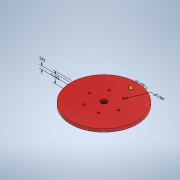
# Autodesk Inventor part: attachementToTripod
Saved by Autodesk Inventor 2022.2 (Build 262287010, 287A)
## iProperties
Created: 2021-02-15
Part Number: attachementToTripod
Material: PC/ABS Plastic
Document SubType Name: Modeling
Designer: robst
Density: 0.357273 g/cm^3
Appearance: Red
Author: robst
Autodesk Inventor part; units mm, degrees
(part 1 of 2)
ref_plane "YZ Plane" through (0, 0, 0) normal (1, 0, 0) x (0, 1, 0)
ref_plane "XZ Plane" through (0, 0, 0) normal (0, 1, 0) x (-1, 0, 0)
ref_plane "XY Plane" through (0, 0, 0) normal (0, 0, 1) x (1, 0, 0)
sketch "Sketch2" plane through (0, 0, 0) normal (0, 0, 1) x (1, 0, 0)
  line L0 (-101.6, 0) -> (-101.6, -9.525)
  line L1 (-101.6, -9.525) -> (-12.7, -9.525)
  line L2 (-10.795, -44.525) -> (0, -44.525)
  line L3 (-101.6, 0) -> (0, 0)
  line L4 (0, 0) -> (0, -44.525) construction
  line L5 (0, 0) -> (0, -44.525)
  line L6 (0, -53.43) -> (0, 8.905) projected
  line L7 (-12.7, -9.525) -> (-10.795, -44.525)
  dimension "d0" = 101.6
  dimension "d3" = 9.525
  dimension "d4" = 35
  dimension "d64" = 10.795
  constraints: 14 end point, 3 vertical, 2 horizontal, 1 perpendicular
  measures "d0" distance from line of L0 L3.end
  measures "d3" distance from line of L1 L3.end
  measures "d4" distance from line of L2.start L1
  measures "d64" horizontal distance of L2.start L3.end
revolve "Revolution1" add sketch "Sketch2" angle 360 about axis through (0, -10, 0) along (0, 1, 0)
sketch "Sketch5" plane through (0, -9.525, 0) normal (0, -1, 0) x (1, 0, 0)
  circle A0 centre (0, 0) radius 76.2 construction
  line L0 (-16.696, -77.6726) -> (-16.6474, -77.6818)
  spline S0 degree 2 poles (-16.6474, -77.6818) (-16.5292, -77.7545) (-16.0721, -77.9292) (-15.8841, -77.9649) knots 0 0 0 1 2 2 2
  spline S1 degree 2 poles (-15.8841, -77.9649) (-15.2895, -78.0777) (-14.6786, -77.6405) (-14.5451, -76.9367) knots 0 0 0 1 2 2 2
  line L1 (-14.5451, -76.9367) -> (-14.5094, -76.7486)
  line L2 (-14.5094, -76.7486) -> (-16.0747, -76.4517)
  line L3 (-16.0747, -76.4517) -> (-15.9262, -75.6691)
  line L4 (-15.9262, -75.6691) -> (-14.3913, -75.9603)
  line L5 (-14.3913, -75.9603) -> (-13.474, -71.125)
  line L6 (-13.474, -71.125) -> (-12.5276, -71.3045)
  line L7 (-12.5276, -71.3045) -> (-13.4449, -76.1398)
  line L8 (-13.4449, -76.1398) -> (-12.8078, -76.2606)
  line L9 (-12.8078, -76.2606) -> (-12.9563, -77.0433)
  line L10 (-12.9563, -77.0433) -> (-13.5933, -76.9224)
  line L11 (-13.5933, -76.9224) -> (-13.629, -77.1105)
  spline S2 degree 2 poles (-13.629, -77.1105) (-13.8201, -78.1176) (-14.9971, -78.9879) (-15.9071, -78.8153) knots 0 0 0 1 2 2 2
  spline S3 degree 2 poles (-15.9071, -78.8153) (-16.168, -78.7658) (-16.6612, -78.6157) (-16.8605, -78.5401) knots 0 0 0 1 2 2 2
  line L12 (-16.8605, -78.5401) -> (-16.696, -77.6726)
  line L13 (-16.8729, -70.3978) -> (-15.9346, -70.6161)
  line L14 (-15.9346, -70.6161) -> (-17.2303, -76.1854)
  line L15 (-17.2303, -76.1854) -> (-18.1686, -75.9671)
  line L16 (-18.1686, -75.9671) -> (-16.8729, -70.3978)
  line L17 (-18.4502, -76.878) -> (-17.3857, -77.1256)
  line L18 (-17.3857, -77.1256) -> (-17.6124, -78.1)
  line L19 (-17.6124, -78.1) -> (-18.6769, -77.8523)
  line L20 (-18.6769, -77.8523) -> (-18.4502, -76.878)
  line L21 (-19.193, -69.801) -> (-18.2625, -70.0502)
  line L22 (-18.2625, -70.0502) -> (-20.3217, -77.7388)
  line L23 (-20.3217, -77.7388) -> (-21.2522, -77.4896)
  line L24 (-21.2522, -77.4896) -> (-19.193, -69.801)
  spline S4 degree 2 poles (-22.8786, -68.5442) (-21.5758, -68.9706) (-20.6221, -70.9005) (-21.0639, -72.2503) knots 0 0 0 1 2 2 2
  spline S5 degree 2 poles (-21.0639, -72.2503) (-21.4979, -73.5767) (-23.4036, -74.6943) (-24.5245, -74.3274) knots 0 0 0 1 2 2 2
  spline S6 degree 2 poles (-24.5245, -74.3274) (-25.0292, -74.1622) (-25.7137, -73.6133) (-25.8995, -73.2082) knots 0 0 0 1 2 2 2
  spline S7 degree 2 poles (-25.8995, -73.2082) (-26.0911, -72.8011) (-26.1083, -71.8014) (-25.8951, -71.1499) knots 0 0 0 1 2 2 2
  line L25 (-25.8951, -71.1499) -> (-25.7318, -70.6511)
  line L26 (-25.7318, -70.6511) -> (-21.97, -71.8823)
  spline S8 degree 2 poles (-21.97, -71.8823) (-21.6607, -70.9374) (-22.283, -69.6227) (-23.1281, -69.3461) knots 0 0 0 1 2 2 2
  spline S9 degree 2 poles (-23.1281, -69.3461) (-23.4274, -69.2482) (-24.0526, -69.193) (-24.3219, -69.2218) knots 0 0 0 1 2 2 2
  spline S10 degree 2 poles (-24.3219, -69.2218) (-24.6068, -69.2585) (-25.0144, -69.3525) (-25.1567, -69.4099) knots 0 0 0 1 2 2 2
  line L27 (-25.1567, -69.4099) -> (-25.2095, -69.3926)
  line L28 (-25.2095, -69.3926) -> (-24.883, -68.395)
  spline S11 degree 2 poles (-24.883, -68.395) (-24.7034, -68.3823) (-24.1607, -68.352) (-23.9556, -68.3606) knots 0 0 0 1 2 2 2
  spline S12 degree 2 poles (-23.9556, -68.3606) (-23.6665, -68.3708) (-23.2073, -68.4366) (-22.8786, -68.5442) knots 0 0 0 1 2 2 2
  spline S13 degree 2 poles (-25.0684, -71.6414) (-25.1776, -72.015) (-25.2017, -72.6049) (-25.1146, -72.8348) knots 0 0 0 1 2 2 2
  spline S14 degree 2 poles (-25.1146, -72.8348) (-25.0233, -73.0921) (-24.5956, -73.4725) (-24.2258, -73.5935) knots 0 0 0 1 2 2 2
  spline S15 degree 2 poles (-24.2258, -73.5935) (-23.862, -73.7126) (-23.2803, -73.6625) (-22.9999, -73.5204) knots 0 0 0 1 2 2 2
  spline S16 degree 2 poles (-22.9999, -73.5204) (-22.7234, -73.3705) (-22.3412, -72.9173) (-22.1986, -72.5807) knots 0 0 0 1 2 2 2
  line L29 (-22.1986, -72.5807) -> (-25.0684, -71.6414)
  line L30 (-27.4155, -67.0006) -> (-26.28, -67.454)
  line L31 (-26.28, -67.454) -> (-26.8205, -68.8074)
  line L32 (-26.8205, -68.8074) -> (-27.956, -68.354)
  line L33 (-27.956, -68.354) -> (-27.4155, -67.0006)
  line L34 (-28.9957, -70.9575) -> (-27.8602, -71.4109)
  line L35 (-27.8602, -71.4109) -> (-28.4007, -72.7643)
  line L36 (-28.4007, -72.7643) -> (-29.5362, -72.3109)
  line L37 (-29.5362, -72.3109) -> (-28.9957, -70.9575)
  spline S17 degree 2 poles (-35.2717, -63.9178) (-35.1275, -63.8965) (-34.6336, -63.8095) (-34.4266, -63.8147) knots 0 0 0 1 2 2 2
  spline S18 degree 2 poles (-34.4266, -63.8147) (-34.1392, -63.8136) (-33.6527, -63.9114) (-33.2711, -64.1144) knots 0 0 0 1 2 2 2
  spline S19 degree 2 poles (-33.2711, -64.1144) (-32.9603, -64.2796) (-32.5234, -64.8127) (-32.4239, -65.1384) knots 0 0 0 1 2 2 2
  spline S20 degree 2 poles (-32.4239, -65.1384) (-32.3323, -65.4528) (-32.4117, -66.1939) (-32.5914, -66.532) knots 0 0 0 1 2 2 2
  spline S21 degree 2 poles (-32.5914, -66.532) (-32.8697, -67.0554) (-33.7056, -67.562) (-34.2985, -67.5196) knots 0 0 0 1 2 2 2
  spline S22 degree 2 poles (-34.2985, -67.5196) (-34.8281, -67.4897) (-36.0623, -67.0223) (-36.7532, -66.7038) knots 0 0 0 1 2 2 2
  line L38 (-36.7532, -66.7038) -> (-36.8401, -66.8674)
  spline S23 degree 2 poles (-36.8401, -66.8674) (-36.9967, -67.1618) (-37.011, -67.6228) (-36.9025, -67.8134) knots 0 0 0 1 2 2 2
  spline S24 degree 2 poles (-36.9025, -67.8134) (-36.7941, -68.0039) (-36.36, -68.3187) (-36.1092, -68.452) knots 0 0 0 1 2 2 2
  spline S25 degree 2 poles (-36.1092, -68.452) (-35.8148, -68.6086) (-34.926, -68.8574) (-34.4381, -68.9) knots 0 0 0 1 2 2 2
  line L39 (-34.4381, -68.9) -> (-34.389, -68.9261)
  line L40 (-34.389, -68.9261) -> (-34.85, -69.793)
  spline S26 degree 2 poles (-34.85, -69.793) (-35.1192, -69.7338) (-36.084, -69.4306) (-36.5147, -69.2015) knots 0 0 0 1 2 2 2
  spline S27 degree 2 poles (-36.5147, -69.2015) (-37.0381, -68.9232) (-37.6654, -68.3799) (-37.8358, -68.0165) knots 0 0 0 1 2 2 2
  spline S28 degree 2 poles (-37.8358, -68.0165) (-38.0037, -67.6614) (-37.9255, -66.8568) (-37.6733, -66.3824) knots 0 0 0 1 2 2 2
  line L41 (-37.6733, -66.3824) -> (-35.8381, -62.9312)
  line L42 (-35.8381, -62.9312) -> (-34.9876, -63.3835)
  line L43 (-34.9876, -63.3835) -> (-35.2717, -63.9178)
  line L44 (-35.6486, -64.6266) -> (-36.3937, -66.0278)
  spline S29 degree 2 poles (-36.3937, -66.0278) (-36.0739, -66.1629) (-35.1032, -66.5601) (-34.7678, -66.6266) knots 0 0 0 1 2 2 2
  spline S30 degree 2 poles (-34.7678, -66.6266) (-34.3747, -66.7027) (-33.704, -66.5068) (-33.5011, -66.1252) knots 0 0 0 1 2 2 2
  spline S31 degree 2 poles (-33.5011, -66.1252) (-33.2692, -65.689) (-33.525, -64.9865) (-33.9939, -64.7371) knots 0 0 0 1 2 2 2
  spline S32 degree 2 poles (-33.9939, -64.7371) (-34.3919, -64.5255) (-35.2288, -64.5211) (-35.6486, -64.6266) knots 0 0 0 1 2 2 2
  spline S33 degree 2 poles (-38.41, -61.232) (-37.7418, -61.6425) (-37.4581, -62.8677) (-37.9656, -63.6937) knots 0 0 0 1 2 2 2
  line L45 (-37.9656, -63.6937) -> (-39.6239, -66.3928)
  line L46 (-39.6239, -66.3928) -> (-39.0715, -66.7322)
  line L47 (-39.0715, -66.7322) -> (-39.4884, -67.4109)
  line L48 (-39.4884, -67.4109) -> (-40.0409, -67.0715)
  line L49 (-40.0409, -67.0715) -> (-40.9007, -68.471)
  line L50 (-40.9007, -68.471) -> (-41.7215, -67.9668)
  line L51 (-41.7215, -67.9668) -> (-40.8617, -66.5673)
  line L52 (-40.8617, -66.5673) -> (-42.3717, -65.6395)
  line L53 (-42.3717, -65.6395) -> (-41.9547, -64.9608)
  line L54 (-41.9547, -64.9608) -> (-40.4447, -65.8885)
  line L55 (-40.4447, -65.8885) -> (-39.0191, -63.5683)
  spline S34 degree 2 poles (-39.0191, -63.5683) (-38.7929, -63.2) (-38.5703, -62.7787) (-38.553, -62.5501) knots 0 0 0 1 2 2 2
  spline S35 degree 2 poles (-38.553, -62.5501) (-38.533, -62.3523) (-38.7707, -61.996) (-39.0548, -61.8215) knots 0 0 0 1 2 2 2
  spline S36 degree 2 poles (-39.0548, -61.8215) (-39.2547, -61.6987) (-39.7026, -61.5902) (-39.8094, -61.5753) knots 0 0 0 1 2 2 2
  line L56 (-39.8094, -61.5753) -> (-39.8568, -61.5462)
  line L57 (-39.8568, -61.5462) -> (-39.4042, -60.8096)
  spline S37 degree 2 poles (-39.4042, -60.8096) (-39.1339, -60.8887) (-38.6152, -61.1059) (-38.41, -61.232) knots 0 0 0 1 2 2 2
  spline S38 degree 2 poles (-41.33, -59.3002) (-40.6824, -59.7426) (-40.4584, -60.9801) (-41.0053, -61.7806) knots 0 0 0 1 2 2 2
  line L58 (-41.0053, -61.7806) -> (-42.7924, -64.3962)
  line L59 (-42.7924, -64.3962) -> (-42.257, -64.762)
  line L60 (-42.257, -64.762) -> (-42.7064, -65.4197)
  line L61 (-42.7064, -65.4197) -> (-43.2417, -65.0539)
  line L62 (-43.2417, -65.0539) -> (-44.1684, -66.4102)
  line L63 (-44.1684, -66.4102) -> (-44.9637, -65.8667)
  line L64 (-44.9637, -65.8667) -> (-44.0371, -64.5105)
  line L65 (-44.0371, -64.5105) -> (-45.5005, -63.5107)
  line L66 (-45.5005, -63.5107) -> (-45.0511, -62.853)
  line L67 (-45.0511, -62.853) -> (-43.5878, -63.8528)
  line L68 (-43.5878, -63.8528) -> (-42.0515, -61.6043)
  spline S39 degree 2 poles (-42.0515, -61.6043) (-41.8077, -61.2474) (-41.565, -60.8373) (-41.5367, -60.6099) knots 0 0 0 1 2 2 2
  spline S40 degree 2 poles (-41.5367, -60.6099) (-41.5071, -60.4132) (-41.7272, -60.0459) (-42.0026, -59.8578) knots 0 0 0 1 2 2 2
  spline S41 degree 2 poles (-42.0026, -59.8578) (-42.1963, -59.7254) (-42.6385, -59.5954) (-42.7444, -59.5753) knots 0 0 0 1 2 2 2
  line L69 (-42.7444, -59.5753) -> (-42.7903, -59.544)
  line L70 (-42.7903, -59.544) -> (-42.3026, -58.8302)
  spline S42 degree 2 poles (-42.3026, -58.8302) (-42.0365, -58.9223) (-41.5288, -59.1644) (-41.33, -59.3002) knots 0 0 0 1 2 2 2
  spline S43 degree 2 poles (-45.7395, -56.8988) (-45.5938, -56.9027) (-45.0923, -56.9019) (-44.8892, -56.9426) knots 0 0 0 1 2 2 2
  spline S44 degree 2 poles (-44.8892, -56.9426) (-44.606, -56.991) (-44.1436, -57.171) (-43.8025, -57.4366) knots 0 0 0 1 2 2 2
  spline S45 degree 2 poles (-43.8025, -57.4366) (-43.5248, -57.6528) (-43.1861, -58.2531) (-43.144, -58.591) knots 0 0 0 1 2 2 2
  spline S46 degree 2 poles (-43.144, -58.591) (-43.1079, -58.9166) (-43.3136, -59.633) (-43.5488, -59.935) knots 0 0 0 1 2 2 2
  spline S47 degree 2 poles (-43.5488, -59.935) (-43.913, -60.4028) (-44.8236, -60.7581) (-45.4003, -60.6143) knots 0 0 0 1 2 2 2
  spline S48 degree 2 poles (-45.4003, -60.6143) (-45.9169, -60.4938) (-47.0522, -59.8211) (-47.6781, -59.3885) knots 0 0 0 1 2 2 2
  line L71 (-47.6781, -59.3885) -> (-47.7919, -59.5347)
  spline S49 degree 2 poles (-47.7919, -59.5347) (-47.9967, -59.7978) (-48.0901, -60.2494) (-48.0161, -60.4558) knots 0 0 0 1 2 2 2
  spline S50 degree 2 poles (-48.0161, -60.4558) (-47.942, -60.6622) (-47.5685, -61.0469) (-47.3444, -61.2215) knots 0 0 0 1 2 2 2
  spline S51 degree 2 poles (-47.3444, -61.2215) (-47.0812, -61.4263) (-46.2485, -61.8243) (-45.7752, -61.9502) knots 0 0 0 1 2 2 2
  line L72 (-45.7752, -61.9502) -> (-45.7314, -61.9843)
  line L73 (-45.7314, -61.9843) -> (-46.3346, -62.759)
  spline S52 degree 2 poles (-46.3346, -62.759) (-46.5896, -62.6544) (-47.4878, -62.1897) (-47.8728, -61.89) knots 0 0 0 1 2 2 2
  spline S53 degree 2 poles (-47.8728, -61.89) (-48.3405, -61.5258) (-48.8649, -60.8827) (-48.9703, -60.4954) knots 0 0 0 1 2 2 2
  spline S54 degree 2 poles (-48.9703, -60.4954) (-49.0747, -60.1168) (-48.8592, -59.3375) (-48.5292, -58.9137) knots 0 0 0 1 2 2 2
  line L74 (-48.5292, -58.9137) -> (-46.1278, -55.8295)
  line L75 (-46.1278, -55.8295) -> (-45.3677, -56.4213)
  line L76 (-45.3677, -56.4213) -> (-45.7395, -56.8988)
  line L77 (-46.2327, -57.5322) -> (-47.2077, -58.7844)
  spline S55 degree 2 poles (-47.2077, -58.7844) (-46.9158, -58.9725) (-46.0279, -59.5308) (-45.709, -59.6539) knots 0 0 0 1 2 2 2
  spline S56 degree 2 poles (-45.709, -59.6539) (-45.3348, -59.7965) (-44.6405, -59.7189) (-44.3749, -59.3778) knots 0 0 0 1 2 2 2
  spline S57 degree 2 poles (-44.3749, -59.3778) (-44.0714, -58.9881) (-44.2026, -58.252) (-44.6217, -57.9257) knots 0 0 0 1 2 2 2
  spline S58 degree 2 poles (-44.6217, -57.9257) (-44.9773, -57.6488) (-45.801, -57.5005) (-46.2327, -57.5322) knots 0 0 0 1 2 2 2
  spline S59 degree 2 poles (-48.7573, -53.3347) (-48.3167, -53.7313) (-47.8308, -54.659) (-47.8171, -55.1698) knots 0 0 0 1 2 2 2
  spline S60 degree 2 poles (-47.8171, -55.1698) (-47.7992, -55.6761) (-48.262, -56.7716) (-48.7661, -57.3315) knots 0 0 0 1 2 2 2
  spline S61 degree 2 poles (-48.7661, -57.3315) (-49.2701, -57.8914) (-50.3038, -58.4398) (-50.8041, -58.4879) knots 0 0 0 1 2 2 2
  spline S62 degree 2 poles (-50.8041, -58.4879) (-51.3086, -58.5406) (-52.3252, -58.1655) (-52.7566, -57.7771) knots 0 0 0 1 2 2 2
  spline S63 degree 2 poles (-52.7566, -57.7771) (-53.1053, -57.4632) (-53.5794, -56.6791) (-53.7161, -56.3234) knots 0 0 0 1 2 2 2
  line L78 (-53.7161, -56.3234) -> (-52.9931, -55.5203)
  line L79 (-52.9931, -55.5203) -> (-52.9518, -55.5575)
  spline S64 degree 2 poles (-52.9518, -55.5575) (-52.9316, -55.6919) (-52.8417, -56.072) (-52.7504, -56.3121) knots 0 0 0 1 2 2 2
  spline S65 degree 2 poles (-52.7504, -56.3121) (-52.6651, -56.5218) (-52.3645, -57.0001) (-52.1809, -57.1654) knots 0 0 0 1 2 2 2
  spline S66 degree 2 poles (-52.1809, -57.1654) (-51.6256, -57.6653) (-50.1949, -57.4328) (-49.5049, -56.6664) knots 0 0 0 1 2 2 2
  spline S67 degree 2 poles (-49.5049, -56.6664) (-48.8315, -55.9183) (-48.7271, -54.4918) (-49.3054, -53.9712) knots 0 0 0 1 2 2 2
  spline S68 degree 2 poles (-49.3054, -53.9712) (-49.6542, -53.6572) (-50.5478, -53.3762) (-50.9935, -53.3821) knots 0 0 0 1 2 2 2
  line L80 (-50.9935, -53.3821) -> (-51.0348, -53.3449)
  line L81 (-51.0348, -53.3449) -> (-50.3118, -52.5418)
  spline S69 degree 2 poles (-50.3118, -52.5418) (-50.1608, -52.5863) (-49.7114, -52.7333) (-49.554, -52.8168) knots 0 0 0 1 2 2 2
  spline S70 degree 2 poles (-49.554, -52.8168) (-49.3209, -52.927) (-48.9822, -53.1322) (-48.7573, -53.3347) knots 0 0 0 1 2 2 2
  line L82 (-53.8319, -48.4518) -> (-53.1654, -49.1473)
  line L83 (-53.1654, -49.1473) -> (-55.5193, -51.4032)
  spline S71 degree 2 poles (-55.5193, -51.4032) (-55.8046, -51.6767) (-56.2438, -52.2001) (-56.314, -52.4214) knots 0 0 0 1 2 2 2
  spline S72 degree 2 poles (-56.314, -52.4214) (-56.3888, -52.6556) (-56.2499, -53.1041) (-56.0021, -53.3626) knots 0 0 0 1 2 2 2
  spline S73 degree 2 poles (-56.0021, -53.3626) (-55.7543, -53.6212) (-54.9523, -53.9047) (-54.4773, -53.9541) knots 0 0 0 1 2 2 2
  line L84 (-54.4773, -53.9541) -> (-51.3922, -50.9974)
  line L85 (-51.3922, -50.9974) -> (-50.7257, -51.6929)
  line L86 (-50.7257, -51.6929) -> (-56.4724, -57.2003)
  line L87 (-56.4724, -57.2003) -> (-57.1389, -56.5048)
  line L88 (-57.1389, -56.5048) -> (-55.0613, -54.5138)
  spline S74 degree 2 poles (-55.0613, -54.5138) (-55.6413, -54.4709) (-56.5123, -54.151) (-56.8371, -53.8122) knots 0 0 0 1 2 2 2
  spline S75 degree 2 poles (-56.8371, -53.8122) (-57.4181, -53.2059) (-57.2736, -51.7502) (-56.5113, -51.0196) knots 0 0 0 1 2 2 2
  line L89 (-56.5113, -51.0196) -> (-53.8319, -48.4518)
  spline S76 degree 2 poles (-56.1935, -45.4316) (-55.3254, -46.4926) (-55.5612, -48.6323) (-56.6604, -49.5317) knots 0 0 0 1 2 2 2
  spline S77 degree 2 poles (-56.6604, -49.5317) (-57.7405, -50.4155) (-59.9481, -50.3308) (-60.695, -49.418) knots 0 0 0 1 2 2 2
  spline S78 degree 2 poles (-60.695, -49.418) (-61.0313, -49.007) (-61.3124, -48.1758) (-61.2507, -47.7344) knots 0 0 0 1 2 2 2
  spline S79 degree 2 poles (-61.2507, -47.7344) (-61.1929, -47.2882) (-60.669, -46.4366) (-60.1385, -46.0026) knots 0 0 0 1 2 2 2
  line L90 (-60.1385, -46.0026) -> (-59.7322, -45.6702)
  line L91 (-59.7322, -45.6702) -> (-57.2257, -48.7336)
  spline S80 degree 2 poles (-57.2257, -48.7336) (-56.4563, -48.104) (-56.2725, -46.6612) (-56.8356, -45.973) knots 0 0 0 1 2 2 2
  spline S81 degree 2 poles (-56.8356, -45.973) (-57.035, -45.7292) (-57.5321, -45.346) (-57.7745, -45.2252) knots 0 0 0 1 2 2 2
  spline S82 degree 2 poles (-57.7745, -45.2252) (-58.0343, -45.1027) (-58.4284, -44.9624) (-58.5792, -44.9342) knots 0 0 0 1 2 2 2
  line L92 (-58.5792, -44.9342) -> (-58.6144, -44.8911)
  line L93 (-58.6144, -44.8911) -> (-57.8019, -44.2264)
  spline S83 degree 2 poles (-57.8019, -44.2264) (-57.6437, -44.3124) (-57.1702, -44.5792) (-57.002, -44.6969) knots 0 0 0 1 2 2 2
  spline S84 degree 2 poles (-57.002, -44.6969) (-56.7639, -44.8611) (-56.4124, -45.164) (-56.1935, -45.4316) knots 0 0 0 1 2 2 2
  spline S85 degree 2 poles (-59.7066, -46.8619) (-59.9999, -47.1178) (-60.3379, -47.6019) (-60.3883, -47.8426) knots 0 0 0 1 2 2 2
  spline S86 degree 2 poles (-60.3883, -47.8426) (-60.45, -48.1085) (-60.2944, -48.6594) (-60.048, -48.9605) knots 0 0 0 1 2 2 2
  spline S87 degree 2 poles (-60.048, -48.9605) (-59.8056, -49.2568) (-59.2886, -49.5279) (-58.9758, -49.5591) knots 0 0 0 1 2 2 2
  spline S88 degree 2 poles (-58.9758, -49.5591) (-58.6621, -49.5817) (-58.0959, -49.4058) (-57.7944, -49.1989) knots 0 0 0 1 2 2 2
  line L94 (-57.7944, -49.1989) -> (-59.7066, -46.8619)
  line L95 (-61.8141, -37.7766) -> (-64.5699, -39.6097)
  spline S89 degree 2 poles (-64.5699, -39.6097) (-64.899, -39.8286) (-65.4252, -40.2528) (-65.5247, -40.4377) knots 0 0 0 1 2 2 2
  spline S90 degree 2 poles (-65.5247, -40.4377) (-65.6396, -40.6328) (-65.5956, -41.0559) (-65.4143, -41.3284) knots 0 0 0 1 2 2 2
  spline S91 degree 2 poles (-65.4143, -41.3284) (-65.2501, -41.5751) (-64.5706, -41.9389) (-64.0843, -42.0456) knots 0 0 0 1 2 2 2
  spline S92 degree 2 poles (-64.0843, -42.0456) (-64.0157, -41.9926) (-63.8221, -41.8489) (-63.6884, -41.76) knots 0 0 0 1 2 2 2
  line L96 (-63.6884, -41.76) -> (-60.5521, -39.6738)
  line L97 (-60.5521, -39.6738) -> (-60.0186, -40.4759)
  line L98 (-60.0186, -40.4759) -> (-62.7744, -42.309)
  spline S93 degree 2 poles (-62.7744, -42.309) (-63.1034, -42.5279) (-63.6297, -42.9521) (-63.7292, -43.1369) knots 0 0 0 1 2 2 2
  spline S94 degree 2 poles (-63.7292, -43.1369) (-63.8441, -43.3321) (-63.8, -43.7551) (-63.6188, -44.0276) knots 0 0 0 1 2 2 2
  spline S95 degree 2 poles (-63.6188, -44.0276) (-63.4478, -44.2847) (-62.7442, -44.6399) (-62.3145, -44.7397) knots 0 0 0 1 2 2 2
  line L99 (-62.3145, -44.7397) -> (-58.7566, -42.3731)
  line L100 (-58.7566, -42.3731) -> (-58.2231, -43.1751)
  line L101 (-58.2231, -43.1751) -> (-62.9841, -46.3421)
  line L102 (-62.9841, -46.3421) -> (-63.5176, -45.54)
  line L103 (-63.5176, -45.54) -> (-62.9931, -45.1911)
  spline S96 degree 2 poles (-62.9931, -45.1911) (-63.5154, -45.0861) (-64.2703, -44.6983) (-64.5165, -44.3281) knots 0 0 0 1 2 2 2
  spline S97 degree 2 poles (-64.5165, -44.3281) (-64.797, -43.9065) (-64.8457, -42.9971) (-64.5215, -42.5367) knots 0 0 0 1 2 2 2
  spline S98 degree 2 poles (-64.5215, -42.5367) (-65.1705, -42.4418) (-66.0453, -42.0299) (-66.312, -41.6289) knots 0 0 0 1 2 2 2
  spline S99 degree 2 poles (-66.312, -41.6289) (-66.5172, -41.3204) (-66.6622, -40.69) (-66.5693, -40.3612) knots 0 0 0 1 2 2 2
  spline S100 degree 2 poles (-66.5693, -40.3612) (-66.4799, -40.0274) (-65.9723, -39.3856) (-65.4839, -39.0607) knots 0 0 0 1 2 2 2
  line L104 (-65.4839, -39.0607) -> (-62.3476, -36.9745)
  line L105 (-62.3476, -36.9745) -> (-61.8141, -37.7766)
  spline S101 degree 2 poles (-64.0171, -33.5193) (-63.3741, -34.73) (-64.0254, -36.7819) (-65.2797, -37.4481) knots 0 0 0 1 2 2 2
  spline S102 degree 2 poles (-65.2797, -37.4481) (-66.5122, -38.1027) (-68.6602, -37.5864) (-69.2134, -36.5447) knots 0 0 0 1 2 2 2
  spline S103 degree 2 poles (-69.2134, -36.5447) (-69.4625, -36.0757) (-69.575, -35.2055) (-69.4279, -34.7848) knots 0 0 0 1 2 2 2
  spline S104 degree 2 poles (-69.4279, -34.7848) (-69.2837, -34.3586) (-68.6028, -33.6264) (-67.9974, -33.3049) knots 0 0 0 1 2 2 2
  line L106 (-67.9974, -33.3049) -> (-67.5339, -33.0588)
  line L107 (-67.5339, -33.0588) -> (-65.6773, -36.5545)
  spline S105 degree 2 poles (-65.6773, -36.5545) (-64.7993, -36.0882) (-64.3359, -34.7095) (-64.753, -33.9241) knots 0 0 0 1 2 2 2
  spline S106 degree 2 poles (-64.753, -33.9241) (-64.9007, -33.646) (-65.3129, -33.1727) (-65.5269, -33.0067) knots 0 0 0 1 2 2 2
  spline S107 degree 2 poles (-65.5269, -33.0067) (-65.7576, -32.8356) (-66.1165, -32.6206) (-66.2588, -32.5634) knots 0 0 0 1 2 2 2
  line L108 (-66.2588, -32.5634) -> (-66.2848, -32.5143)
  line L109 (-66.2848, -32.5143) -> (-65.3577, -32.0219)
  spline S108 degree 2 poles (-65.3577, -32.0219) (-65.2195, -32.1373) (-64.8075, -32.4918) (-64.6657, -32.6403) knots 0 0 0 1 2 2 2
  spline S109 degree 2 poles (-64.6657, -32.6403) (-64.4645, -32.848) (-64.1793, -33.2139) (-64.0171, -33.5193) knots 0 0 0 1 2 2 2
  spline S110 degree 2 poles (-67.7426, -34.2324) (-68.0804, -34.4258) (-68.5068, -34.834) (-68.6035, -35.0601) knots 0 0 0 1 2 2 2
  spline S111 degree 2 poles (-68.6035, -35.0601) (-68.7162, -35.3088) (-68.6718, -35.8795) (-68.4893, -36.2231) knots 0 0 0 1 2 2 2
  spline S112 degree 2 poles (-68.4893, -36.2231) (-68.3097, -36.5612) (-67.856, -36.9285) (-67.5554, -37.0206) knots 0 0 0 1 2 2 2
  spline S113 degree 2 poles (-67.5554, -37.0206) (-67.2522, -37.1043) (-66.6626, -37.0428) (-66.3263, -36.8992) knots 0 0 0 1 2 2 2
  line L110 (-66.3263, -36.8992) -> (-67.7426, -34.2324)
  line L111 (-67.2989, -26.7639) -> (-66.9151, -27.6475)
  line L112 (-66.9151, -27.6475) -> (-69.9055, -28.9465)
  spline S114 degree 2 poles (-69.9055, -28.9465) (-70.268, -29.104) (-70.8615, -29.4426) (-71.0041, -29.6257) knots 0 0 0 1 2 2 2
  spline S115 degree 2 poles (-71.0041, -29.6257) (-71.1556, -29.8195) (-71.1809, -30.2882) (-71.0382, -30.6167) knots 0 0 0 1 2 2 2
  spline S116 degree 2 poles (-71.0382, -30.6167) (-70.8955, -30.9452) (-70.2417, -31.4893) (-69.8133, -31.7005) knots 0 0 0 1 2 2 2
  line L113 (-69.8133, -31.7005) -> (-65.894, -29.9979)
  line L114 (-65.894, -29.9979) -> (-65.5102, -30.8815)
  line L115 (-65.5102, -30.8815) -> (-70.7548, -33.1597)
  line L116 (-70.7548, -33.1597) -> (-71.1386, -32.2762)
  line L117 (-71.1386, -32.2762) -> (-70.5553, -32.0228)
  spline S117 degree 2 poles (-70.5553, -32.0228) (-71.0843, -31.7813) (-71.7903, -31.1791) (-71.9773, -30.7487) knots 0 0 0 1 2 2 2
  spline S118 degree 2 poles (-71.9773, -30.7487) (-72.3119, -29.9784) (-71.6713, -28.6633) (-70.7028, -28.2426) knots 0 0 0 1 2 2 2
  line L118 (-70.7028, -28.2426) -> (-67.2989, -26.7639)
  spline S119 degree 2 poles (-68.2413, -23.8288) (-67.9759, -24.5667) (-68.5196, -25.7007) (-69.4318, -26.0288) knots 0 0 0 1 2 2 2
  line L119 (-69.4318, -26.0288) -> (-72.4127, -27.1009)
  line L120 (-72.4127, -27.1009) -> (-72.1933, -27.711)
  line L121 (-72.1933, -27.711) -> (-72.9428, -27.9806)
  line L122 (-72.9428, -27.9806) -> (-73.1623, -27.3705)
  line L123 (-73.1623, -27.3705) -> (-74.7079, -27.9264)
  line L124 (-74.7079, -27.9264) -> (-75.0339, -27.02)
  line L125 (-75.0339, -27.02) -> (-73.4883, -26.464)
  line L126 (-73.4883, -26.464) -> (-74.0881, -24.7964)
  line L127 (-74.0881, -24.7964) -> (-73.3385, -24.5268)
  line L128 (-73.3385, -24.5268) -> (-72.7387, -26.1945)
  line L129 (-72.7387, -26.1945) -> (-70.1762, -25.2728)
  spline S120 degree 2 poles (-70.1762, -25.2728) (-69.7695, -25.1265) (-69.3325, -24.9365) (-69.1763, -24.7688) knots 0 0 0 1 2 2 2
  spline S121 degree 2 poles (-69.1763, -24.7688) (-69.037, -24.6268) (-69.0002, -24.2002) (-69.113, -23.8864) knots 0 0 0 1 2 2 2
  spline S122 degree 2 poles (-69.113, -23.8864) (-69.1925, -23.6656) (-69.4745, -23.3011) (-69.5486, -23.2228) knots 0 0 0 1 2 2 2
  line L130 (-69.5486, -23.2228) -> (-69.5674, -23.1705)
  line L131 (-69.5674, -23.1705) -> (-68.7539, -22.8779)
  spline S123 degree 2 poles (-68.7539, -22.8779) (-68.5922, -23.1085) (-68.3228, -23.6022) (-68.2413, -23.8288) knots 0 0 0 1 2 2 2
  line L132 (-69.4547, -20.4114) -> (-75.9138, -22.2601)
  line L133 (-75.9138, -22.2601) -> (-75.2103, -24.7178)
  line L134 (-75.2103, -24.7178) -> (-76.0771, -24.9659)
  line L135 (-76.0771, -24.9659) -> (-77.7626, -19.0767)
  line L136 (-77.7626, -19.0767) -> (-76.8958, -18.8287)
  line L137 (-76.8958, -18.8287) -> (-76.1924, -21.2864)
  line L138 (-76.1924, -21.2864) -> (-69.7333, -19.4378)
  line L139 (-69.7333, -19.4378) -> (-69.4547, -20.4114)
  spline S124 degree 2 poles (-74.2908, -12.2398) (-72.8739, -11.9567) (-71.0575, -13.0106) (-70.8301, -14.149) knots 0 0 0 1 2 2 2
  spline S125 degree 2 poles (-70.8301, -14.149) (-70.5966, -15.3177) (-71.9217, -16.9741) (-73.2902, -17.2476) knots 0 0 0 1 2 2 2
  spline S126 degree 2 poles (-73.2902, -17.2476) (-74.6951, -17.5283) (-76.5272, -16.4586) (-76.7522, -15.3323) knots 0 0 0 1 2 2 2
  spline S127 degree 2 poles (-76.7522, -15.3323) (-76.9797, -14.1939) (-75.7017, -12.5217) (-74.2908, -12.2398) knots 0 0 0 1 2 2 2
  spline S128 degree 2 poles (-74.096, -13.2147) (-75.186, -13.4325) (-76.0872, -14.4375) (-75.9408, -15.1702) knots 0 0 0 1 2 2 2
  spline S129 degree 2 poles (-75.9408, -15.1702) (-75.7944, -15.9029) (-74.575, -16.4904) (-73.485, -16.2727) knots 0 0 0 1 2 2 2
  spline S130 degree 2 poles (-73.485, -16.2727) (-72.4253, -16.0609) (-71.4951, -15.0438) (-71.6415, -14.3111) knots 0 0 0 1 2 2 2
  spline S131 degree 2 poles (-71.6415, -14.3111) (-71.7867, -13.5845) (-73.0182, -12.9993) (-74.096, -13.2147) knots 0 0 0 1 2 2 2
  line L140 (-71.8472, -8.8632) -> (-78.5207, -9.6385)
  line L141 (-78.5207, -9.6385) -> (-78.2257, -12.1779)
  line L142 (-78.2257, -12.1779) -> (-79.1213, -12.2819)
  line L143 (-79.1213, -12.2819) -> (-79.8282, -6.1972)
  line L144 (-79.8282, -6.1972) -> (-78.9326, -6.0932)
  line L145 (-78.9326, -6.0932) -> (-78.6376, -8.6326)
  line L146 (-78.6376, -8.6326) -> (-71.9641, -7.8572)
  line L147 (-71.9641, -7.8572) -> (-71.8472, -8.8632)
  line L148 (-77.0777, -1.8047) -> (-77.0754, -1.8541)
  spline S132 degree 2 poles (-77.0754, -1.8541) (-77.1009, -1.9665) (-77.1019, -2.2077) (-77.094, -2.3742) knots 0 0 0 1 2 2 2
  spline S133 degree 2 poles (-77.094, -2.3742) (-77.0756, -2.7628) (-76.7002, -3.5116) (-76.3508, -3.8413) knots 0 0 0 1 2 2 2
  line L149 (-76.3508, -3.8413) -> (-72.2983, -3.6495)
  line L150 (-72.2983, -3.6495) -> (-72.2528, -4.6118)
  line L151 (-72.2528, -4.6118) -> (-77.9645, -4.882)
  line L152 (-77.9645, -4.882) -> (-78.01, -3.9198)
  line L153 (-78.01, -3.9198) -> (-77.1588, -3.8795)
  spline S134 degree 2 poles (-77.1588, -3.8795) (-77.6524, -3.3774) (-78.0719, -2.6121) (-78.0894, -2.242) knots 0 0 0 1 2 2 2
  spline S135 degree 2 poles (-78.0894, -2.242) (-78.0964, -2.094) (-78.0911, -1.9454) (-78.0769, -1.852) knots 0 0 0 1 2 2 2
  line L154 (-78.0769, -1.852) -> (-77.0777, -1.8047)
  line L155 (-72.3915, 0.146) -> (-72.387, -0.8173)
  line L156 (-72.387, -0.8173) -> (-78.105, -0.8438)
  line L157 (-78.105, -0.8438) -> (-78.1095, 0.1195)
  line L158 (-78.1095, 0.1195) -> (-72.3915, 0.146)
  line L159 (-79.0607, 0.183) -> (-79.0557, -0.9099)
  line L160 (-79.0557, -0.9099) -> (-80.056, -0.9146)
  line L161 (-80.056, -0.9146) -> (-80.0611, 0.1784)
  line L162 (-80.0611, 0.1784) -> (-79.0607, 0.183)
  spline S136 degree 2 poles (-75.1674, 6.5014) (-73.7367, 6.4271) (-72.1178, 4.9765) (-72.1719, 3.9343) knots 0 0 0 1 2 2 2
  spline S137 degree 2 poles (-72.1719, 3.9343) (-72.194, 3.5088) (-72.4253, 2.8654) (-72.6464, 2.5368) knots 0 0 0 1 2 2 2
  line L163 (-72.6464, 2.5368) -> (-70.2537, 2.4125)
  line L164 (-70.2537, 2.4125) -> (-70.3037, 1.4505)
  line L165 (-70.3037, 1.4505) -> (-78.117, 1.8564)
  line L166 (-78.117, 1.8564) -> (-78.067, 2.8184)
  line L167 (-78.067, 2.8184) -> (-77.4688, 2.7873)
  spline S138 degree 2 poles (-77.4688, 2.7873) (-77.7771, 3.162) (-78.1633, 4.0601) (-78.1367, 4.5719) knots 0 0 0 1 2 2 2
  spline S139 degree 2 poles (-78.1367, 4.5719) (-78.0857, 5.5524) (-76.4747, 6.5694) (-75.1674, 6.5014) knots 0 0 0 1 2 2 2
  spline S140 degree 2 poles (-75.1079, 5.5028) (-76.0884, 5.5538) (-77.2, 4.987) (-77.2362, 4.2901) knots 0 0 0 1 2 2 2
  spline S141 degree 2 poles (-77.2362, 4.2901) (-77.2573, 3.8831) (-76.9332, 3.0996) (-76.6671, 2.7457) knots 0 0 0 1 2 2 2
  line L168 (-76.6671, 2.7457) -> (-73.4234, 2.5772)
  spline S142 degree 2 poles (-73.4234, 2.5772) (-73.2251, 2.9441) (-73.0615, 3.4735) (-73.0436, 3.8189) knots 0 0 0 1 2 2 2
  spline S143 degree 2 poles (-73.0436, 3.8189) (-73.0048, 4.565) (-74.0596, 5.4484) (-75.1079, 5.5028) knots 0 0 0 1 2 2 2
  spline S144 degree 2 poles (-74.269, 12.3716) (-72.8364, 12.1827) (-71.457, 10.5993) (-71.6088, 9.4484) knots 0 0 0 1 2 2 2
  spline S145 degree 2 poles (-71.6088, 9.4484) (-71.7647, 8.2668) (-73.5532, 7.1262) (-74.9368, 7.3087) knots 0 0 0 1 2 2 2
  spline S146 degree 2 poles (-74.9368, 7.3087) (-76.3571, 7.4961) (-77.7463, 9.0994) (-77.5961, 10.2381) knots 0 0 0 1 2 2 2
  spline S147 degree 2 poles (-77.5961, 10.2381) (-77.4443, 11.389) (-75.6954, 12.5598) (-74.269, 12.3716) knots 0 0 0 1 2 2 2
  spline S148 degree 2 poles (-74.399, 11.386) (-75.5009, 11.5313) (-76.6781, 10.8707) (-76.7758, 10.1299) knots 0 0 0 1 2 2 2
  spline S149 degree 2 poles (-76.7758, 10.1299) (-76.8735, 9.3891) (-75.9087, 8.4397) (-74.8068, 8.2944) knots 0 0 0 1 2 2 2
  spline S150 degree 2 poles (-74.8068, 8.2944) (-73.7354, 8.153) (-72.5269, 8.8158) (-72.4292, 9.5566) knots 0 0 0 1 2 2 2
  spline S151 degree 2 poles (-72.4292, 9.5566) (-72.3323, 10.2912) (-73.3093, 11.2422) (-74.399, 11.386) knots 0 0 0 1 2 2 2
  line L169 (-70.3347, 17.2679) -> (-70.5358, 16.3258)
  line L170 (-70.5358, 16.3258) -> (-71.1035, 16.4471)
  spline S152 degree 2 poles (-71.1035, 16.4471) (-70.9687, 16.191) (-70.7955, 15.8193) (-70.7393, 15.58) knots 0 0 0 1 2 2 2
  spline S153 degree 2 poles (-70.7393, 15.58) (-70.6852, 15.3601) (-70.6741, 14.9094) (-70.7348, 14.6256) knots 0 0 0 1 2 2 2
  spline S154 degree 2 poles (-70.7348, 14.6256) (-70.8328, 14.1666) (-71.3783, 13.4749) (-71.8047, 13.2818) knots 0 0 0 1 2 2 2
  spline S155 degree 2 poles (-71.8047, 13.2818) (-72.2311, 13.0887) (-73.3826, 13.0189) (-74.0891, 13.1698) knots 0 0 0 1 2 2 2
  spline S156 degree 2 poles (-74.0891, 13.1698) (-74.8259, 13.3271) (-75.8195, 13.9371) (-76.1532, 14.3557) knots 0 0 0 1 2 2 2
  spline S157 degree 2 poles (-76.1532, 14.3557) (-76.4498, 14.741) (-76.682, 15.6936) (-76.5802, 16.1707) knots 0 0 0 1 2 2 2
  spline S158 degree 2 poles (-76.5802, 16.1707) (-76.4912, 16.5873) (-76.1711, 17.1694) (-75.9044, 17.4723) knots 0 0 0 1 2 2 2
  line L171 (-75.9044, 17.4723) -> (-78.3199, 17.9882)
  line L172 (-78.3199, 17.9882) -> (-78.1188, 18.9302)
  line L173 (-78.1188, 18.9302) -> (-70.3347, 17.2679)
  line L174 (-71.8946, 16.616) -> (-75.1254, 17.306)
  spline S159 degree 2 poles (-75.1254, 17.306) (-75.3693, 16.9918) (-75.6147, 16.4633) (-75.6831, 16.1432) knots 0 0 0 1 2 2 2
  spline S160 degree 2 poles (-75.6831, 16.1432) (-75.8378, 15.4186) (-74.9262, 14.3652) (-73.8996, 14.1459) knots 0 0 0 1 2 2 2
  spline S161 degree 2 poles (-73.8996, 14.1459) (-72.9092, 13.9344) (-71.7304, 14.3394) (-71.5821, 15.0339) knots 0 0 0 1 2 2 2
  spline S162 degree 2 poles (-71.5821, 15.0339) (-71.5034, 15.4022) (-71.6817, 16.2233) (-71.8946, 16.616) knots 0 0 0 1 2 2 2
  line L175 (-69.5601, 20.0516) -> (-69.8889, 18.874)
  line L176 (-69.8889, 18.874) -> (-71.2926, 19.266)
  line L177 (-71.2926, 19.266) -> (-70.9637, 20.4436)
  line L178 (-70.9637, 20.4436) -> (-69.5601, 20.0516)
  line L179 (-68.7753, 22.5943) -> (-69.0699, 21.6771)
  line L180 (-69.0699, 21.6771) -> (-74.5141, 23.4256)
  line L181 (-74.5141, 23.4256) -> (-74.2195, 24.3428)
  line L182 (-74.2195, 24.3428) -> (-68.7753, 22.5943)
  line L183 (-75.1041, 24.6982) -> (-75.4384, 23.6576)
  line L184 (-75.4384, 23.6576) -> (-76.3908, 23.9635)
  line L185 (-76.3908, 23.9635) -> (-76.0566, 25.0041)
  line L186 (-76.0566, 25.0041) -> (-75.1041, 24.6982)
  spline S163 degree 2 poles (-69.4429, 29.4973) (-68.1058, 28.9828) (-67.0168, 27.1016) (-67.3915, 26.1276) knots 0 0 0 1 2 2 2
  spline S164 degree 2 poles (-67.3915, 26.1276) (-67.5445, 25.73) (-67.964, 25.19) (-68.2761, 24.9462) knots 0 0 0 1 2 2 2
  line L187 (-68.2761, 24.9462) -> (-66.04, 24.0859)
  line L188 (-66.04, 24.0859) -> (-66.3859, 23.1868)
  line L189 (-66.3859, 23.1868) -> (-73.6879, 25.9963)
  line L190 (-73.6879, 25.9963) -> (-73.3419, 26.8953)
  line L191 (-73.3419, 26.8953) -> (-72.7829, 26.6802)
  spline S165 degree 2 poles (-72.7829, 26.6802) (-72.9598, 27.132) (-73.0483, 28.1056) (-72.8643, 28.584) knots 0 0 0 1 2 2 2
  spline S166 degree 2 poles (-72.8643, 28.584) (-72.5117, 29.5003) (-70.6647, 29.9674) (-69.4429, 29.4973) knots 0 0 0 1 2 2 2
  spline S167 degree 2 poles (-69.6961, 28.5295) (-70.6125, 28.8821) (-71.845, 28.688) (-72.0956, 28.0368) knots 0 0 0 1 2 2 2
  spline S168 degree 2 poles (-72.0956, 28.0368) (-72.2419, 27.6564) (-72.1768, 26.8109) (-72.0337, 26.392) knots 0 0 0 1 2 2 2
  line L192 (-72.0337, 26.392) -> (-69.0023, 25.2256)
  spline S169 degree 2 poles (-69.0023, 25.2256) (-68.6999, 25.5129) (-68.3802, 25.9655) (-68.256, 26.2882) knots 0 0 0 1 2 2 2
  spline S170 degree 2 poles (-68.256, 26.2882) (-67.9877, 26.9856) (-68.7164, 28.1525) (-69.6961, 28.5295) knots 0 0 0 1 2 2 2
  spline S171 degree 2 poles (-65.3722, 30.8409) (-65.7002, 30.1286) (-66.8828, 29.701) (-67.7634, 30.1064) knots 0 0 0 1 2 2 2
  line L193 (-67.7634, 30.1064) -> (-70.6409, 31.4313)
  line L194 (-70.6409, 31.4313) -> (-70.912, 30.8424)
  line L195 (-70.912, 30.8424) -> (-71.6356, 31.1755)
  line L196 (-71.6356, 31.1755) -> (-71.3644, 31.7645)
  line L197 (-71.3644, 31.7645) -> (-72.8564, 32.4514)
  line L198 (-72.8564, 32.4514) -> (-72.4535, 33.3264)
  line L199 (-72.4535, 33.3264) -> (-70.9615, 32.6395)
  line L200 (-70.9615, 32.6395) -> (-70.2203, 34.2493)
  line L201 (-70.2203, 34.2493) -> (-69.4968, 33.9161)
  line L202 (-69.4968, 33.9161) -> (-70.238, 32.3063)
  line L203 (-70.238, 32.3063) -> (-67.7644, 31.1674)
  spline S172 degree 2 poles (-67.7644, 31.1674) (-67.3718, 30.9866) (-66.9269, 30.8158) (-66.6979, 30.8259) knots 0 0 0 1 2 2 2
  spline S173 degree 2 poles (-66.6979, 30.8259) (-66.4991, 30.8295) (-66.1738, 31.108) (-66.0343, 31.4109) knots 0 0 0 1 2 2 2
  spline S174 degree 2 poles (-66.0343, 31.4109) (-65.9362, 31.624) (-65.8818, 32.0817) (-65.8797, 32.1895) knots 0 0 0 1 2 2 2
  line L204 (-65.8797, 32.1895) -> (-65.8565, 32.24)
  line L205 (-65.8565, 32.24) -> (-65.0712, 31.8784)
  spline S175 degree 2 poles (-65.0712, 31.8784) (-65.1176, 31.6006) (-65.2715, 31.0597) (-65.3722, 30.8409) knots 0 0 0 1 2 2 2
  spline S176 degree 2 poles (-61.9264, 37.1541) (-62.2187, 36.667) (-62.9896, 36.0422) (-63.4281, 35.9235) knots 0 0 0 1 2 2 2
  spline S177 degree 2 poles (-63.4281, 35.9235) (-63.858, 35.807) (-64.7497, 35.9532) (-65.1574, 36.1978) knots 0 0 0 1 2 2 2
  spline S178 degree 2 poles (-65.1574, 36.1978) (-65.6869, 36.5155) (-66.2366, 37.6158) (-66.1773, 38.3147) knots 0 0 0 1 2 2 2
  line L206 (-66.1773, 38.3147) -> (-66.2038, 38.3306)
  spline S179 degree 2 poles (-66.2038, 38.3306) (-66.7735, 38.0171) (-67.7203, 37.9515) (-68.218, 38.2501) knots 0 0 0 1 2 2 2
  spline S180 degree 2 poles (-68.218, 38.2501) (-68.954, 38.6917) (-69.2718, 40.3946) (-68.7571, 41.2524) knots 0 0 0 1 2 2 2
  spline S181 degree 2 poles (-68.7571, 41.2524) (-68.2234, 42.142) (-66.6465, 42.6577) (-65.9158, 42.2193) knots 0 0 0 1 2 2 2
  spline S182 degree 2 poles (-65.9158, 42.2193) (-65.4763, 41.9556) (-64.9267, 40.9273) (-64.9722, 40.2993) knots 0 0 0 1 2 2 2
  line L207 (-64.9722, 40.2993) -> (-64.9457, 40.2835)
  spline S183 degree 2 poles (-64.9457, 40.2835) (-64.3378, 40.6965) (-63.2227, 40.8268) (-62.6191, 40.4646) knots 0 0 0 1 2 2 2
  spline S184 degree 2 poles (-62.6191, 40.4646) (-61.7824, 39.9626) (-61.38, 38.0649) (-61.9264, 37.1541) knots 0 0 0 1 2 2 2
  spline S185 degree 2 poles (-63.0744, 39.5136) (-63.4768, 39.755) (-64.144, 39.7233) (-64.6576, 39.4193) knots 0 0 0 1 2 2 2
  spline S186 degree 2 poles (-64.6576, 39.4193) (-64.8313, 39.3219) (-65.3259, 38.9417) (-65.6404, 38.7055) knots 0 0 0 1 2 2 2
  spline S187 degree 2 poles (-65.6404, 38.7055) (-65.6181, 38.2025) (-65.1405, 37.3902) (-64.6904, 37.1202) knots 0 0 0 1 2 2 2
  spline S188 degree 2 poles (-64.6904, 37.1202) (-64.0974, 36.7644) (-62.8954, 37.0154) (-62.5713, 37.5555) knots 0 0 0 1 2 2 2
  spline S189 degree 2 poles (-62.5713, 37.5555) (-62.2409, 38.1062) (-62.5025, 39.1705) (-63.0744, 39.5136) knots 0 0 0 1 2 2 2
  spline S190 degree 2 poles (-66.4199, 41.3551) (-66.8594, 41.6188) (-67.7998, 41.3837) (-68.1143, 40.8595) knots 0 0 0 1 2 2 2
  spline S191 degree 2 poles (-68.1143, 40.8595) (-68.4002, 40.3829) (-68.2413, 39.4595) (-67.7912, 39.1894) knots 0 0 0 1 2 2 2
  spline S192 degree 2 poles (-67.7912, 39.1894) (-67.4682, 38.9956) (-66.8307, 39.038) (-66.4632, 39.2424) knots 0 0 0 1 2 2 2
  spline S193 degree 2 poles (-66.4632, 39.2424) (-66.3097, 39.3303) (-65.7135, 39.7359) (-65.5027, 39.9191) knots 0 0 0 1 2 2 2
  spline S194 degree 2 poles (-65.5027, 39.9191) (-65.5652, 40.4751) (-66.0227, 41.1169) (-66.4199, 41.3551) knots 0 0 0 1 2 2 2
  line L208 (-65.0379, 47.2065) -> (-62.7337, 45.3288)
  line L209 (-62.7337, 45.3288) -> (-63.1187, 44.7767)
  line L210 (-63.1187, 44.7767) -> (-65.6772, 46.2897)
  line L211 (-65.6772, 46.2897) -> (-65.0379, 47.2065)
  line L212 (-66.1398, 45.6262) -> (-63.8357, 43.7485)
  line L213 (-63.8357, 43.7485) -> (-64.2207, 43.1964)
  line L214 (-64.2207, 43.1964) -> (-66.7791, 44.7094)
  line L215 (-66.7791, 44.7094) -> (-66.1398, 45.6262)
  line L216 (-52.8185, 49.5515) -> (-53.456, 48.8292)
  line L217 (-53.456, 48.8292) -> (-53.8912, 49.2134)
  spline S195 degree 2 poles (-53.8912, 49.2134) (-53.8994, 48.9241) (-53.9308, 48.5153) (-53.9992, 48.2791) knots 0 0 0 1 2 2 2
  spline S196 degree 2 poles (-53.9992, 48.2791) (-54.0599, 48.061) (-54.2714, 47.6628) (-54.4634, 47.4452) knots 0 0 0 1 2 2 2
  spline S197 degree 2 poles (-54.4634, 47.4452) (-54.774, 47.0934) (-55.5887, 46.7582) (-56.055, 46.7991) knots 0 0 0 1 2 2 2
  spline S198 degree 2 poles (-56.055, 46.7991) (-56.5213, 46.8401) (-57.5589, 47.3441) (-58.1006, 47.8222) knots 0 0 0 1 2 2 2
  spline S199 degree 2 poles (-58.1006, 47.8222) (-58.6654, 48.3207) (-59.232, 49.3398) (-59.3175, 49.8682) knots 0 0 0 1 2 2 2
  spline S200 degree 2 poles (-59.3175, 49.8682) (-59.3869, 50.3495) (-59.122, 51.2934) (-58.7992, 51.6592) knots 0 0 0 1 2 2 2
  spline S201 degree 2 poles (-58.7992, 51.6592) (-58.5172, 51.9786) (-57.9528, 52.3288) (-57.5717, 52.4619) knots 0 0 0 1 2 2 2
  line L218 (-57.5717, 52.4619) -> (-59.4236, 54.0964)
  line L219 (-59.4236, 54.0964) -> (-58.7861, 54.8187)
  line L220 (-58.7861, 54.8187) -> (-52.8185, 49.5515)
  line L221 (-54.4977, 49.7487) -> (-56.9745, 51.9348)
  spline S202 degree 2 poles (-56.9745, 51.9348) (-57.3411, 51.7807) (-57.8143, 51.4406) (-58.0309, 51.1952) knots 0 0 0 1 2 2 2
  spline S203 degree 2 poles (-58.0309, 51.1952) (-58.5212, 50.6397) (-58.2436, 49.2745) (-57.4566, 48.5798) knots 0 0 0 1 2 2 2
  spline S204 degree 2 poles (-57.4566, 48.5798) (-56.6973, 47.9097) (-55.4714, 47.6842) (-55.0015, 48.2167) knots 0 0 0 1 2 2 2
  spline S205 degree 2 poles (-55.0015, 48.2167) (-54.7522, 48.4991) (-54.5048, 49.302) (-54.4977, 49.7487) knots 0 0 0 1 2 2 2
  line L222 (-51.1413, 51.2359) -> (-51.8185, 50.5508)
  line L223 (-51.8185, 50.5508) -> (-55.8849, 54.5709)
  line L224 (-55.8849, 54.5709) -> (-55.2076, 55.256)
  line L225 (-55.2076, 55.256) -> (-51.1413, 51.2359)
  line L226 (-55.8362, 55.9728) -> (-56.6046, 55.1956)
  line L227 (-56.6046, 55.1956) -> (-57.316, 55.8989)
  line L228 (-57.316, 55.8989) -> (-56.5476, 56.6761)
  line L229 (-56.5476, 56.6761) -> (-55.8362, 55.9728)
  spline S206 degree 2 poles (-48.1966, 54.833) (-48.2254, 54.6902) (-48.3108, 54.196) (-48.3858, 54.0029) knots 0 0 0 1 2 2 2
  spline S207 degree 2 poles (-48.3858, 54.0029) (-48.4821, 53.7322) (-48.7389, 53.3076) (-49.0591, 53.0172) knots 0 0 0 1 2 2 2
  spline S208 degree 2 poles (-49.0591, 53.0172) (-49.3198, 52.7808) (-49.9693, 52.5502) (-50.3095, 52.5668) knots 0 0 0 1 2 2 2
  spline S209 degree 2 poles (-50.3095, 52.5668) (-50.6364, 52.5872) (-51.3068, 52.9128) (-51.564, 53.1964) knots 0 0 0 1 2 2 2
  spline S210 degree 2 poles (-51.564, 53.1964) (-51.9622, 53.6355) (-52.1559, 54.5936) (-51.9151, 55.1371) knots 0 0 0 1 2 2 2
  spline S211 degree 2 poles (-51.9151, 55.1371) (-51.7077, 55.6253) (-50.8499, 56.6282) (-50.3163, 57.1705) knots 0 0 0 1 2 2 2
  line L230 (-50.3163, 57.1705) -> (-50.4408, 57.3077)
  spline S212 degree 2 poles (-50.4408, 57.3077) (-50.6648, 57.5547) (-51.0937, 57.7243) (-51.3097, 57.6868) knots 0 0 0 1 2 2 2
  spline S213 degree 2 poles (-51.3097, 57.6868) (-51.5258, 57.6492) (-51.9689, 57.3474) (-52.1793, 57.1565) knots 0 0 0 1 2 2 2
  spline S214 degree 2 poles (-52.1793, 57.1565) (-52.4263, 56.9325) (-52.9614, 56.1805) (-53.1668, 55.7359) knots 0 0 0 1 2 2 2
  line L231 (-53.1668, 55.7359) -> (-53.2079, 55.6986)
  line L232 (-53.2079, 55.6986) -> (-53.8675, 56.4259)
  spline S215 degree 2 poles (-53.8675, 56.4259) (-53.7206, 56.6591) (-53.1086, 57.4642) (-52.7472, 57.7919) knots 0 0 0 1 2 2 2
  spline S216 degree 2 poles (-52.7472, 57.7919) (-52.3081, 58.1902) (-51.5844, 58.5964) (-51.1848, 58.6337) knots 0 0 0 1 2 2 2
  spline S217 degree 2 poles (-51.1848, 58.6337) (-50.7939, 58.6714) (-50.0632, 58.3253) (-49.7023, 57.9274) knots 0 0 0 1 2 2 2
  line L233 (-49.7023, 57.9274) -> (-47.0765, 55.0319)
  line L234 (-47.0765, 55.0319) -> (-47.7901, 54.3848)
  line L235 (-47.7901, 54.3848) -> (-48.1966, 54.833)
  line L236 (-48.7359, 55.4277) -> (-49.802, 56.6033)
  spline S218 degree 2 poles (-49.802, 56.6033) (-50.0374, 56.3481) (-50.7399, 55.5693) (-50.916, 55.2762) knots 0 0 0 1 2 2 2
  spline S219 degree 2 poles (-50.916, 55.2762) (-51.1208, 54.9321) (-51.1636, 54.2348) (-50.8732, 53.9146) knots 0 0 0 1 2 2 2
  spline S220 degree 2 poles (-50.8732, 53.9146) (-50.5413, 53.5486) (-49.7936, 53.5515) (-49.4003, 53.9082) knots 0 0 0 1 2 2 2
  spline S221 degree 2 poles (-49.4003, 53.9082) (-49.0663, 54.211) (-48.7788, 54.997) (-48.7359, 55.4277) knots 0 0 0 1 2 2 2
  line L237 (-40.8747, 59.8106) -> (-42.8457, 62.4695)
  spline S222 degree 2 poles (-42.8457, 62.4695) (-43.0811, 62.787) (-43.5315, 63.291) (-43.7212, 63.381) knots 0 0 0 1 2 2 2
  spline S223 degree 2 poles (-43.7212, 63.381) (-43.9219, 63.4858) (-44.3422, 63.4202) (-44.6051, 63.2253) knots 0 0 0 1 2 2 2
  spline S224 degree 2 poles (-44.6051, 63.2253) (-44.8432, 63.0488) (-45.172, 62.3516) (-45.2537, 61.8606) knots 0 0 0 1 2 2 2
  spline S225 degree 2 poles (-45.2537, 61.8606) (-45.1973, 61.7948) (-45.044, 61.6087) (-44.9483, 61.4797) knots 0 0 0 1 2 2 2
  line L238 (-44.9483, 61.4797) -> (-42.7052, 58.4537)
  line L239 (-42.7052, 58.4537) -> (-43.479, 57.88)
  line L240 (-43.479, 57.88) -> (-45.4501, 60.5389)
  spline S226 degree 2 poles (-45.4501, 60.5389) (-45.6854, 60.8564) (-46.1359, 61.3604) (-46.3256, 61.4504) knots 0 0 0 1 2 2 2
  spline S227 degree 2 poles (-46.3256, 61.4504) (-46.5263, 61.5552) (-46.9466, 61.4896) (-47.2095, 61.2947) knots 0 0 0 1 2 2 2
  spline S228 degree 2 poles (-47.2095, 61.2947) (-47.4575, 61.1109) (-47.7765, 60.3902) (-47.8542, 59.9559) knots 0 0 0 1 2 2 2
  line L241 (-47.8542, 59.9559) -> (-45.3095, 56.5231)
  line L242 (-45.3095, 56.5231) -> (-46.0834, 55.9494)
  line L243 (-46.0834, 55.9494) -> (-49.4886, 60.543)
  line L244 (-49.4886, 60.543) -> (-48.7147, 61.1167)
  line L245 (-48.7147, 61.1167) -> (-48.3397, 60.6107)
  spline S229 degree 2 poles (-48.3397, 60.6107) (-48.2614, 61.1376) (-47.9125, 61.9112) (-47.5553, 62.176) knots 0 0 0 1 2 2 2
  spline S230 degree 2 poles (-47.5553, 62.176) (-47.1485, 62.4776) (-46.2427, 62.5725) (-45.7664, 62.2722) knots 0 0 0 1 2 2 2
  spline S231 degree 2 poles (-45.7664, 62.2722) (-45.7047, 62.9252) (-45.3379, 63.8198) (-44.9509, 64.1066) knots 0 0 0 1 2 2 2
  spline S232 degree 2 poles (-44.9509, 64.1066) (-44.6533, 64.3273) (-44.0311, 64.5041) (-43.6981, 64.4281) knots 0 0 0 1 2 2 2
  spline S233 degree 2 poles (-43.6981, 64.4281) (-43.3601, 64.3558) (-42.6933, 63.8816) (-42.344, 63.4103) knots 0 0 0 1 2 2 2
  line L246 (-42.344, 63.4103) -> (-40.1008, 60.3843)
  line L247 (-40.1008, 60.3843) -> (-40.8747, 59.8106)
  line L248 (-37.6488, 61.8324) -> (-38.6878, 61.1878)
  line L249 (-38.6878, 61.1878) -> (-39.456, 62.4262)
  line L250 (-39.456, 62.4262) -> (-38.4171, 63.0707)
  line L251 (-38.4171, 63.0707) -> (-37.6488, 61.8324)
  spline S234 degree 2 poles (-31.249, 71.2044) (-31.0349, 70.7592) (-30.9667, 69.8053) (-31.1167, 69.3906) knots 0 0 0 1 2 2 2
  spline S235 degree 2 poles (-31.1167, 69.3906) (-31.3043, 68.8687) (-32.0931, 68.044) (-32.8277, 67.6907) knots 0 0 0 1 2 2 2
  line L252 (-32.8277, 67.6907) -> (-33.6012, 67.3187)
  line L253 (-33.6012, 67.3187) -> (-32.3701, 64.7589)
  line L254 (-32.3701, 64.7589) -> (-33.2827, 64.32)
  line L255 (-33.2827, 64.32) -> (-36.5853, 71.1871)
  line L256 (-36.5853, 71.1871) -> (-34.8601, 72.0168)
  spline S236 degree 2 poles (-34.8601, 72.0168) (-34.248, 72.3111) (-33.2946, 72.523) (-32.8566, 72.4527) knots 0 0 0 1 2 2 2
  spline S237 degree 2 poles (-32.8566, 72.4527) (-32.3468, 72.3758) (-31.5247, 71.7776) (-31.249, 71.2044) knots 0 0 0 1 2 2 2
  spline S238 degree 2 poles (-32.1873, 70.719) (-32.3585, 71.0751) (-32.855, 71.4805) (-33.1857, 71.527) knots 0 0 0 1 2 2 2
  spline S239 degree 2 poles (-33.1857, 71.527) (-33.4723, 71.5673) (-34.1073, 71.4058) (-34.5358, 71.1998) knots 0 0 0 1 2 2 2
  line L257 (-34.5358, 71.1998) -> (-35.2926, 70.8358)
  line L258 (-35.2926, 70.8358) -> (-33.9759, 68.0978)
  line L259 (-33.9759, 68.0978) -> (-33.3526, 68.3976)
  spline S240 degree 2 poles (-33.3526, 68.3976) (-32.7961, 68.6652) (-32.1972, 69.1725) (-32.087, 69.5132) knots 0 0 0 1 2 2 2
  spline S241 degree 2 poles (-32.087, 69.5132) (-31.9802, 69.8182) (-32.0294, 70.3906) (-32.1873, 70.719) knots 0 0 0 1 2 2 2
  line L260 (-25.6067, 75.8662) -> (-25.3416, 67.8113)
  line L261 (-25.3416, 67.8113) -> (-26.3627, 67.4216)
  line L262 (-26.3627, 67.4216) -> (-31.5317, 73.6049)
  line L263 (-31.5317, 73.6049) -> (-30.5163, 73.9924)
  line L264 (-30.5163, 73.9924) -> (-26.2864, 68.8321)
  line L265 (-26.2864, 68.8321) -> (-26.5702, 75.4985)
  line L266 (-26.5702, 75.4985) -> (-25.6067, 75.8662)
  spline S242 degree 2 poles (-18.8132, 73.8814) (-18.244, 71.9118) (-18.8557, 69.736) (-20.0481, 69.3914) knots 0 0 0 1 2 2 2
  spline S243 degree 2 poles (-20.0481, 69.3914) (-21.2583, 69.0417) (-22.9348, 70.5947) (-23.492, 72.5227) knots 0 0 0 1 2 2 2
  spline S244 degree 2 poles (-23.492, 72.5227) (-24.0646, 74.5041) (-23.4495, 76.6681) (-22.2512, 77.0144) knots 0 0 0 1 2 2 2
  spline S245 degree 2 poles (-22.2512, 77.0144) (-21.0469, 77.3624) (-19.3652, 75.7915) (-18.8132, 73.8814) knots 0 0 0 1 2 2 2
  spline S246 degree 2 poles (-19.4262, 71.2874) (-19.3884, 71.6904) (-19.592, 72.8399) (-19.8098, 73.5933) knots 0 0 0 1 2 2 2
  spline S247 degree 2 poles (-19.8098, 73.5933) (-20.0275, 74.3467) (-20.4668, 75.4218) (-20.7231, 75.7526) knots 0 0 0 1 2 2 2
  spline S248 degree 2 poles (-20.7231, 75.7526) (-20.9794, 76.0835) (-21.6069, 76.3199) (-22.0163, 76.2017) knots 0 0 0 1 2 2 2
  spline S249 degree 2 poles (-22.0163, 76.2017) (-22.4256, 76.0834) (-22.8421, 75.5452) (-22.8849, 75.115) knots 0 0 0 1 2 2 2
  spline S250 degree 2 poles (-22.8849, 75.115) (-22.9252, 74.6984) (-22.7028, 73.5285) (-22.4954, 72.8107) knots 0 0 0 1 2 2 2
  spline S251 degree 2 poles (-22.4954, 72.8107) (-22.2725, 72.0395) (-21.8793, 71.0348) (-21.6084, 70.6759) knots 0 0 0 1 2 2 2
  spline S252 degree 2 poles (-21.6084, 70.6759) (-21.3563, 70.3374) (-20.7101, 70.0807) (-20.283, 70.2041) knots 0 0 0 1 2 2 2
  spline S253 degree 2 poles (-20.283, 70.2041) (-19.8796, 70.3207) (-19.463, 70.8589) (-19.4262, 71.2874) knots 0 0 0 1 2 2 2
  line L267 (-12.5309, 73.9998) -> (-13.4201, 73.8173)
  line L268 (-13.4201, 73.8173) -> (-12.8938, 71.2525)
  line L269 (-12.8938, 71.2525) -> (-13.8556, 71.0552)
  line L270 (-13.8556, 71.0552) -> (-14.3819, 73.62)
  line L271 (-14.3819, 73.62) -> (-17.6786, 72.9435)
  line L272 (-17.6786, 72.9435) -> (-17.8946, 73.996)
  line L273 (-17.8946, 73.996) -> (-15.345, 78.5283)
  line L274 (-15.345, 78.5283) -> (-14.4255, 78.717)
  line L275 (-14.4255, 78.717) -> (-13.5852, 74.6218)
  line L276 (-13.5852, 74.6218) -> (-12.696, 74.8043)
  line L277 (-12.696, 74.8043) -> (-12.5309, 73.9998)
  line L278 (-14.547, 74.4245) -> (-15.1453, 77.3401)
  line L279 (-15.1453, 77.3401) -> (-17.0573, 73.9093)
  line L280 (-17.0573, 73.9093) -> (-14.547, 74.4245)